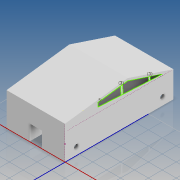
# Autodesk Inventor part: prototype 2
Saved by Autodesk Inventor 2020 (Build 240168000, 168)
## iProperties
Created: 2019-12-03
Part Number: prototype 2
Material: Generic
Document SubType Name: Modeling
Designer: Berkant
Density: 1 g/cm^3
Appearance: Default
Author: Berkant
Autodesk Inventor part; units mm, degrees
ref_plane "YZ Plane" through (0, 0, 0) normal (1, 0, 0) x (0, 1, 0)
ref_plane "XZ Plane" through (0, 0, 0) normal (0, 1, 0) x (-1, 0, 0)
ref_plane "XY Plane" through (0, 0, 0) normal (0, 0, 1) x (1, 0, 0)
sketch "Sketch1" plane through (0, 0, 0) normal (0, 1, 0) x (-1, 0, 0)
  line L0 (0, 0) -> (84, 0)
  line L1 (84, 0) -> (84, -156)
  line L2 (84, -156) -> (0, -156)
  line L3 (0, -156) -> (0, 0)
  line L4 (84, 0) -> (84, -3)
  line L5 (84, -3) -> (81, -3) construction
  line L6 (0, -156) -> (0, -153)
  line L7 (0, -153) -> (3, -153) construction
  line L8 (81, -3) -> (3, -3)
  line L9 (3, -3) -> (3, -153)
  line L10 (3, -153) -> (81, -153)
  line L11 (81, -153) -> (81, -3)
  dimension "d0" = 84
  dimension "d1" = 156
  dimension "d2" = 3
  dimension "d3" = 3
  dimension "d4" = 3
  dimension "d5" = 3
  constraints: 24 end point, 4 parallel, 4 perpendicular, 2 horizontal, 2 point on line
  measures "d0" distance of L1.end L2.end
  measures "d1" distance of L0.end L1.end
  measures "d2" distance of L0.end L4.end
  measures "d3" distance of L4.end L5.end
  measures "d4" distance of L2.end L6.end
  measures "d5" distance of L6.end L7.end
extrude "Extrusion1" add sketch "Sketch1" along normal blind 15 contours L0 L1 L2 L3 | L11 L10 L9 L8
sketch "Sketch2" plane through (0, 15, 0) normal (0, 1, 0) x (1, 0, 0)
  line L0 (-84, 156) -> (-84, 0) projected
  line L1 (-84, 0) -> (-84, 3)
  line L2 (-84, 3) -> (-81, 3) construction
  line L3 (0, 0) -> (0, 156) projected
  line L4 (0, 156) -> (0, 153)
  line L5 (0, 153) -> (-3, 153) construction
  line L6 (-81, 3) -> (-3, 3)
  line L7 (-3, 3) -> (-3, 153)
  line L8 (-3, 153) -> (-81, 153)
  line L9 (-81, 153) -> (-81, 3)
  dimension "d8" = 3
  dimension "d9" = 3
  dimension "d10" = 3
  dimension "d11" = 3
  constraints: 16 end point, 3 perpendicular, 2 parallel, 2 point on line, 1 horizontal
  measures "d8" distance of L0.end L1.end
  measures "d9" distance of L1.end L2.end
  measures "d10" distance of L3.end L4.end
  measures "d11" distance of L4.end L5.end
extrude "Extrusion2" cut sketch "Sketch2" against normal blind 12
sketch "Sketch15" plane through (-81, 3, -3) normal (1, 0, 0) x (0, 0, -1)
  line L0 (87.2546, 33.7556) -> (153, 12)
  line L1 (153, 12) -> (150, 12)
  line L2 (153, 12) -> (-3, 12)
  line L3 (-3, 12) -> (153, 12) projected
  line L4 (-3, 12) -> (-3, 22)
  line L5 (87.2546, 33.7556) -> (-3, 22)
  dimension "d125" = 10
  constraints: 10 end point, 1 collinear, 1 vertical
  measures "d125" distance of L2.end L4.end
extrude "Extrusion12" add sketch "Sketch15" along normal blind 81 and the other way blind 3
sketch "Sketch16" plane through (0, 0, 0) normal (0, -1, 0) x (1, 0, 0)
  line L0 (0, -156) -> (-3, -156)
  line L1 (0, -153) -> (0, -156)
  line L2 (-3, -153) -> (-30, -153)
  line L3 (-30, -153) -> (-30, -83)
  line L4 (-30, -83) -> (-3, -83)
  line L5 (-3, -83) -> (-3, -153)
  line L6 (-81, -153) -> (-54, -153)
  line L7 (-54, -153) -> (-54, -83)
  line L8 (-54, -83) -> (-81, -83)
  line L9 (-81, -83) -> (-81, -153)
  line L10 (-3, -3) -> (-30, -3)
  line L11 (-30, -3) -> (-30, -73)
  line L12 (-30, -73) -> (-3, -73)
  line L13 (-3, -73) -> (-3, -3)
  line L14 (-81, -3) -> (-53.9385, -3)
  line L15 (-53.9385, -3) -> (-53.9385, -72.9998)
  line L16 (-53.9385, -72.9998) -> (-81, -72.9998)
  line L17 (-81, -72.9998) -> (-81, -3)
  line L18 (-33, -83) -> (-33, -80)
  line L19 (-33, -73) -> (-33, -76)
  line L20 (0, -156) -> (-33, -156)
  line L21 (-33, -156) -> (-33, -80)
  line L22 (0, -80) -> (0, -156)
  line L23 (-84, -156) -> (-51, -156)
  line L24 (-84, -80) -> (-84, -156)
  line L25 (0, 0) -> (-33, 0)
  line L26 (-33, 0) -> (-33, -76)
  line L27 (0, -76) -> (0, 0)
  line L28 (-84, 0) -> (-51, 0)
  line L29 (-51, 0) -> (-51, -72.9998)
  line L30 (-84, -76) -> (-84, 0)
  line L31 (-33, -80) -> (-33, -76)
  line L32 (0, -80) -> (0, -76)
  line L33 (0, -90.2546) -> (0, 0) projected
  line L34 (-51, -156) -> (-51, -83)
  line L35 (-51, -83) -> (-51, -72.9998)
  line L36 (-84, -80) -> (-84, -76)
  line L37 (-84, -156) -> (-84, 0) projected
  constraints: 72 end point, 12 parallel, 9 horizontal, 7 perpendicular, 3 collinear, 2 vertical
extrude "Extrusion13" add sketch "Sketch16" along normal blind 22.5
sketch "Sketch17" plane through (0, -22.5, 0) normal (1, 0, 0) x (0, 0, -1)
  line L0 (156, 22.5) -> (0, 22.5) projected
  line L1 (0, 22.5) -> (16, 22.5)
  line L2 (16, 22.5) -> (16, 11.3)
  line L3 (156, 22.5) -> (156, 0) projected
  line L4 (156, 22.5) -> (140, 22.5)
  line L5 (140, 22.5) -> (140, 11.3)
  circle A0 centre (140, 11.3) radius 3
  circle A1 centre (16, 11.3) radius 3
  dimension "d152" = 16
  dimension "d153" = 11.2
  dimension "d154" = 16
  dimension "d155" = 11.2
  dimension "d156" = 6
  dimension "d157" = 6
  constraints: 8 end point, 2 centre point, 2 coincident, 2 point on line, 1 perpendicular, 1 vertical
  measures "d152" distance of L0.end L1.end
  measures "d153" distance of L1.end L2.end
  measures "d154" distance of L0.start L4.end
  measures "d155" distance of L4.end L5.end
  measures "d156" diameter of A0
  measures "d157" diameter of A1
extrude "Extrusion14" cut sketch "Sketch17" against normal blind 104.25
sketch "Sketch18" plane through (-30, 0, -3) normal (1, 0, 0) x (0, 0, -1)
  circle A0 centre (13, -11.2) radius 3 projected
  line L0 (13, -11.2) -> (63, -11.2)
  circle A1 centre (63, -11.2) radius 1.5
  circle A2 centre (137, -11.2) radius 3 projected
  line L1 (137, -11.2) -> (87, -11.2)
  circle A3 centre (87, -11.2) radius 1.5
  point P0 (-3, 0)
  dimension "d160" = 50
  dimension "d161" = 3
  dimension "d162" = 50
  dimension "d163" = 3
  constraints: 4 end point, 2 centre point, 2 coincident, 2 horizontal
  measures "d160" distance of L0.start L0.end
  measures "d161" diameter of A1
  measures "d162" distance of L1.start L1.end
  measures "d163" diameter of A3
extrude "Extrusion15" cut sketch "Sketch18" against normal blind 35 contours A1 | A3
sketch "Sketch19" plane through (0, -22.5, 0) normal (1, 0, 0) x (0, 0, -1)
  line L0 (24.5867, 50.7024) -> (27.5867, 50.7024) construction
  line L1 (52.4457, 51.3057) -> (87.4417, 55.8638)
  line L2 (87.4417, 55.8638) -> (89.8555, 56.1782)
  line L3 (128.3377, 43.444) -> (89.8555, 56.1782)
  line L4 (128.3377, 43.444) -> (137.0302, 40.5676)
  line L5 (3, 37.5) -> (153, 37.5) construction
  line L6 (136.0152, 37.5) -> (139.0152, 37.5) construction
  line L7 (138.3236, 37.5) -> (141.3236, 37.5) construction
  line L8 (137.0302, 40.5676) -> (139.5212, 39.7465)
  line L9 (0, 47.5) -> (0, 0) construction
  line L10 (139.5212, 39.7465) -> (52.4457, 44.5852)
  line L11 (82.6373, 55.2381) -> (79.6624, 54.8506) construction
  line L12 (82.6373, 55.2381) -> (83.3756, 42.7599)
  line L13 (82.6373, 55.2381) -> (79.6624, 54.8506)
  line L14 (79.6624, 54.8506) -> (80.3616, 43.0339)
  line L15 (119.7308, 46.2922) -> (120.0541, 40.8283)
  line L16 (122.5789, 45.3497) -> (122.8556, 40.6726)
  line L17 (52.4457, 51.3057) -> (47.4876, 50.6599)
  line L18 (47.4876, 50.6599) -> (47.4876, 44.8607)
  line L19 (52.4457, 44.5852) -> (47.4876, 44.8607)
  point P0 (0, 22.5)
  point P1 (83.3692, 42.8668)
  dimension "d178" = 3
  dimension "d180" = 3
  dimension "d182" = 3
  dimension "d183" = 3
  dimension "d184" = 5
  constraints: 36 end point, 9 point on line, 3 horizontal, 2 parallel, 1 vertical
  measures "d178" distance of L11.start L11.end
  measures "d180" distance of L11.start L11.end
  measures "d182" distance of L16.start L15.start
  measures "d183" distance of L16.start L15.start
  measures "d184" distance of L1.start L17.end
extrude "Extrusion17" cut sketch "Sketch19" against normal up to surface (84 mm away) contours L1 L14 L10 L19 L18 L17 | L1 L2 L3 L15 L10 L12 | L16 L3 L4 L8 L10
extrude "Extrusion18" add sketch "Sketch19" along normal blind 0.1 and the other way blind 84.1 contours L1 L14 L10 L19 L18 L17 | L1 L2 L3 L15 L10 L12 | L16 L3 L4 L8 L10
body "Solid1"
